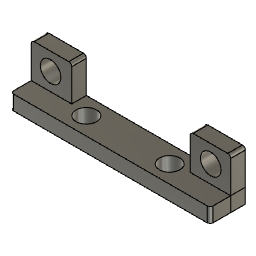
USB-Holder (Autodesk Fusion 360 design; units mm, degrees)
Autodesk Fusion 360 part; units mm, degrees
sketch "Sketch1" plane through (0, 0, 0) normal (0, 0, 1) x (1, 0, 0)
  line L0 (0, 0) -> (34, 0)
  line L1 (34, 0) -> (34, 6)
  line L2 (34, 6) -> (0, 6)
  line L3 (0, 6) -> (0, 0)
  line L4 (17, 6) -> (17, 0) construction
  circle A0 centre (9.9, 3) radius 1.75
  circle A1 centre (24.1, 3) radius 1.75
  line L5 (6.9, 6) -> (6.9, 0)
  line L6 (27.1, 6) -> (27.1, 0)
  line L7 (0, 3.5) -> (6.9, 3.5)
  line L8 (34, 3.5) -> (27.1, 3.5)
  dimension "d2" = 6
  dimension "d3" = 3.5
  dimension "d4" = 7.1
  dimension "d6" = 3
  dimension "d11" = 10.1
  dimension "d13" = 2.5
  dimension "d30" = 17
  constraint horizontal L0
  constraint vertical L1
  constraint horizontal L2
  constraint vertical L3
  constraint coincident L0.start L3.end
  constraint midpoint L2 L4.start
  constraint midpoint L0 L4.end
  constraint symmetric L4 A0 A1
  constraint coincident L2 L5.start
  constraint coincident L0 L5.end
  constraint perpendicular L0 L5
  constraint symmetric L4 L5.start L6.start
  constraint symmetric L4 L5.end L6.end
  constraint coincident L3 L7.start
  constraint coincident L5 L7.end
  constraint perpendicular L5 L7
  constraint symmetric L4 L7.start L8.start
  constraint symmetric L4 L7.end L8.end
  measures "d2" distance of L0.start L2.end
  measures "d3" diameter of A0
  measures "d4" distance of L4 A0.centre
  measures "d6" distance of L0 A0.centre
  measures "d11" distance of L4 L5
  measures "d13" distance of L2 L7
  measures "d30" distance of L3 L4
extrude "Extrude4" add sketch "Sketch1" along normal blind 8.5 contours L2 L3 L5 L7 | L1 L2 L6 L8 makes body 1 at (4.6, 6, 2.8333) makes body 2 at (31.7, 3.5, 2.8333)
extrude "Extrude1" add sketch "Sketch1" along normal blind 2.5 separate body makes body 3
split "Split1" by bodies 3 bodies 1 makes body 4 at (2.3, 3.5, 4.5)
split "Split2" by plane through (0, 0, 2.5) normal (0, 0, 1) bodies 2 makes body 5 at (31.7, 3.5, 4.5)
sketch "Sketch5" plane through (0, 3.5, 0) normal (0, -1, 0) x (1, 0, 0)
  line L0 (0, 2.5) -> (6.9, 2.5)
  line L1 (6.9, 2.5) -> (6.9, 8.5)
  line L2 (6.9, 8.5) -> (0, 8.5)
  line L3 (0, 8.5) -> (0, 2.5)
  circle A0 centre (3.3095, 5.4882) radius 1.75
  circle A1 centre (30.6059, 5.4872) radius 1.75
  line L4 (0, 5.5) -> (6.9, 5.5) construction
  dimension "d22" = 3.5
  dimension "d24" = 3.5
  constraint midpoint L3 L4.start
  constraint midpoint L1 L4.end
  measures "d22" diameter of A0
  measures "d24" diameter of A1
extrude "Extrude5" cut sketch "Sketch5" against normal up to surface (2.5 mm away) contours A0 | A1 bodies 4 5
fillet "Fillet1" radius 0.5 6 edges at (34, 0, 1.25) (0, 0, 1.25) (0, 4.75, 8.5) (6.9, 4.75, 8.5) (27.1, 4.75, 8.5) (34, 4.75, 8.5) on bodies 3 4 5
equation "d2 = Tiefe"
equation "d3 = 3.2 mm + CutoutMargin"
equation "Tiefe = 6 mm"
equation "d6 = Tiefe / 2"
equation "Breite = 17 mm"
equation "d8 = Dicke"
equation "Dicke = 2.5 mm"
equation "d20 = Dicke + 6 mm"
equation "d22 = 3.2 mm + CutoutMargin"
equation "d24 = 3.2 mm + CutoutMargin"
equation "CutoutMargin = 0.3 mm"
equation "d30 = Breite"
